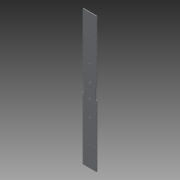
# Autodesk Inventor part: bienal - final pieza superior
Saved by Autodesk Inventor 2015 (Build 190159000, 159)
## iProperties
Created: 2017-03-17
Part Number: bienal - final pieza superior
Material: Generic
Document SubType Name: Modeling
Designer: maxil
Density: 1 g/cm^3
Appearance: Default
Author: maxil
Autodesk Inventor part; units mm, degrees
ref_plane "YZ Plane" through (0, 0, 0) normal (1, 0, 0) x (0, 1, 0)
ref_plane "XZ Plane" through (0, 0, 0) normal (0, 1, 0) x (-1, 0, 0)
ref_plane "XY Plane" through (0, 0, 0) normal (0, 0, 1) x (1, 0, 0)
sketch "Sketch1" plane through (0, 0, 0) normal (0, 1, 0) x (-1, 0, 0)
  line L0 (-28, -290) -> (28, -290)
  line L1 (28, 290) -> (-28, 290)
  line L2 (25, -24.5) -> (30, -24.5)
  line L3 (30, 24.5) -> (25, 24.5)
  line L4 (25, 24.5) -> (25, -24.5)
  line L5 (30, -288) -> (30, -24.5)
  line L6 (30, 24.5) -> (30, 288)
  line L7 (-25, -24.5) -> (-30, -24.5)
  line L8 (-30, 24.5) -> (-25, 24.5)
  line L9 (-25, 24.5) -> (-25, -24.5)
  line L10 (-30, 288) -> (-30, 24.5)
  line L11 (-30, -24.5) -> (-30, -288)
  line L12 (0, 0) -> (0, 200) construction
  circle A0 centre (0, 200) radius 1.5
  line L13 (-30, 200) -> (-20, 200) construction
  circle A1 centre (-20, 200) radius 1.5
  circle A2 centre (20, 200) radius 1.5
  circle A3 centre (0, -200) radius 1.5
  circle A4 centre (-20, -200) radius 1.5
  circle A5 centre (20, -200) radius 1.5
  arc A6 (30, 288) -> (28, 290) centre (28, 288) ccw
  arc A7 (-28, 290) -> (-30, 288) centre (-28, 288) ccw
  arc A8 (28, -290) -> (30, -288) centre (28, -288) ccw
  arc A9 (-30, -288) -> (-28, -290) centre (-28, -288) ccw
  line L14 (25, 0) -> (-25, 0) construction
  circle A10 centre (0, 30) radius 4
  circle A11 centre (0, 100) radius 3
  line L15 (0, 0) -> (0, -200) construction
  circle A12 centre (0, -30) radius 4
  circle A13 centre (0, -100) radius 3
  point P0 (30, 290)
  point P1 (30, -290)
  point P2 (-30, 290)
  dimension "d0" = 60
  dimension "d1" = 580
  dimension "d16" = 200
  dimension "d17" = 3
  dimension "d18" = 10
  dimension "d19" = 2
  dimension "d20" = 2
  dimension "d21" = 2
  dimension "d27" = 8
  dimension "d28" = 6
  dimension "d29" = 60
  constraints: 32 end point, 14 centre point, 9 point on line, 8 point on circle, 8 tangent, 6 coincident, 6 parallel, 5 symmetric about line, 3 horizontal, 3 midpoint, 2 perpendicular, 1 equal radius, 1 vertical, 3 other
  measures "d0" distance of point (-30, 290) point (30, 290)
  measures "d1" distance of point (30, 290) point (30, -290)
  measures "d16" distance of L12.start L12.end
  measures "d17" diameter of A0
  measures "d18" distance of L13.start L13.end
  measures "d19" radius of A6
  measures "d20" radius of A7
  measures "d21" radius of A8
  measures "d27" diameter of A10
  measures "d28" diameter of A11
  measures "d29" distance of A12.centre A10.centre
extrude "Extrusion1" add sketch "Sketch1" along normal blind 3
body "Solid1"
